Autodesk Fusion 360 part; units mm, degrees
(part 7 of 7)
  spline S38 degree 5 poles (-2.0348, 11.0912) (-2.0357, 11.0961) (-2.0377, 11.106) (-2.041, 11.1207) (-2.046, 11.1401) (-2.0533, 11.1642) (-2.0612, 11.1881) (-2.0696, 11.2119) (-2.0783, 11.2357) (-2.0871, 11.2594) (-2.096, 11.2831) (-2.1052, 11.3068) (-2.1147, 11.3304) (-2.1244, 11.3539) (-2.1346, 11.3774) (-2.145, 11.4007) (-2.1557, 11.424) (-2.1666, 11.4472) (-2.1777, 11.4704) (-2.189, 11.4935) (-2.2005, 11.5166) (-2.2122, 11.5397) (-2.2241, 11.5626) (-2.2361, 11.5855) (-2.2484, 11.6084) (-2.2609, 11.6312) (-2.2736, 11.654) (-2.2864, 11.6767) (-2.2995, 11.6993) (-2.3126, 11.7219) (-2.326, 11.7444) (-2.3395, 11.7669) (-2.3532, 11.7894) (-2.3671, 11.8118) (-2.3811, 11.8341) (-2.3953, 11.8564) (-2.4096, 11.8786) (-2.4241, 11.9008) (-2.4387, 11.9229) (-2.4535, 11.945) (-2.4685, 11.967) (-2.4836, 11.989) (-2.4988, 12.011) (-2.5142, 12.0328) (-2.5297, 12.0547) (-2.5454, 12.0764) (-2.5612, 12.0982) (-2.5771, 12.1198) (-2.5932, 12.1415) (-2.6094, 12.163) (-2.6258, 12.1846) (-2.6423, 12.206) (-2.6589, 12.2274) (-2.6756, 12.2488) (-2.6925, 12.2701) (-2.7095, 12.2914) (-2.7267, 12.3126) (-2.744, 12.3338) (-2.7614, 12.3549) (-2.7789, 12.3759) (-2.7965, 12.3969) (-2.8143, 12.4179) (-2.8322, 12.4388) (-2.8502, 12.4596) (-2.8684, 12.4804) (-2.8866, 12.5012) (-2.905, 12.5219) (-2.9235, 12.5425) (-2.9421, 12.5631) (-2.9609, 12.5836) (-2.9797, 12.6041) (-2.9949, 12.6204) (-3.0064, 12.6327) (-3.014, 12.6408) (-3.0178, 12.6449) knots 0 0 0 0 0 0 0.01428571 0.02857143 0.04285714 0.05714286 0.07142857 0.08571429 0.1 0.11428571 0.12857143 0.14285714 0.15714286 0.17142857 0.18571429 0.2 0.21428571 0.22857143 0.24285714 0.25714286 0.27142857 0.28571429 0.3 0.31428571 0.32857143 0.34285714 0.35714286 0.37142857 0.38571429 0.4 0.41428571 0.42857143 0.44285714 0.45714286 0.47142857 0.48571429 0.5 0.51428571 0.52857143 0.54285714 0.55714286 0.57142857 0.58571429 0.6 0.61428571 0.62857143 0.64285714 0.65714286 0.67142857 0.68571429 0.7 0.71428571 0.72857143 0.74285714 0.75714286 0.77142857 0.78571429 0.8 0.81428571 0.82857143 0.84285714 0.85714286 0.87142857 0.88571429 0.9 0.91428571 0.92857143 0.94285714 0.95714286 0.97142857 0.98571429 1 1 1 1 1 1
  arc A39 (-3.0178, 12.6449) -> (-3.7089, 12.4597) centre (0, 0) ccw
  spline S39 degree 5 poles (-3.7089, 12.4597) (-3.7102, 12.4543) (-3.7127, 12.4434) (-3.7165, 12.4271) (-3.7215, 12.4053) (-3.7276, 12.3782) (-3.7336, 12.351) (-3.7394, 12.3239) (-3.7451, 12.2968) (-3.7507, 12.2696) (-3.7561, 12.2426) (-3.7614, 12.2155) (-3.7666, 12.1884) (-3.7717, 12.1614) (-3.7766, 12.1343) (-3.7814, 12.1073) (-3.786, 12.0803) (-3.7905, 12.0533) (-3.7949, 12.0264) (-3.7992, 11.9994) (-3.8033, 11.9725) (-3.8072, 11.9456) (-3.8111, 11.9187) (-3.8147, 11.8919) (-3.8183, 11.865) (-3.8217, 11.8382) (-3.825, 11.8114) (-3.8281, 11.7846) (-3.831, 11.7579) (-3.8339, 11.7312) (-3.8365, 11.7045) (-3.8391, 11.6778) (-3.8415, 11.6512) (-3.8437, 11.6246) (-3.8458, 11.598) (-3.8477, 11.5714) (-3.8495, 11.5449) (-3.8511, 11.5184) (-3.8525, 11.492) (-3.8538, 11.4656) (-3.855, 11.4392) (-3.8559, 11.4128) (-3.8567, 11.3865) (-3.8574, 11.3602) (-3.8578, 11.334) (-3.8581, 11.3078) (-3.8583, 11.2816) (-3.8582, 11.2555) (-3.858, 11.2294) (-3.8576, 11.2034) (-3.857, 11.1774) (-3.8562, 11.1514) (-3.8552, 11.1256) (-3.854, 11.0997) (-3.8526, 11.0739) (-3.851, 11.0482) (-3.8492, 11.0225) (-3.8473, 10.9969) (-3.8451, 10.9713) (-3.8427, 10.9458) (-3.8401, 10.9204) (-3.8371, 10.895) (-3.8339, 10.8698) (-3.8302, 10.8446) (-3.8264, 10.8195) (-3.8223, 10.7945) (-3.818, 10.7695) (-3.8136, 10.7446) (-3.809, 10.7198) (-3.8039, 10.6951) (-3.7981, 10.6706) (-3.7928, 10.6513) (-3.7883, 10.6369) (-3.7851, 10.6274) (-3.7834, 10.6227) knots -1 -1 -1 -1 -1 -1 -0.98571429 -0.97142857 -0.95714286 -0.94285714 -0.92857143 -0.91428571 -0.9 -0.88571429 -0.87142857 -0.85714286 -0.84285714 -0.82857143 -0.81428571 -0.8 -0.78571429 -0.77142857 -0.75714286 -0.74285714 -0.72857143 -0.71428571 -0.7 -0.68571429 -0.67142857 -0.65714286 -0.64285714 -0.62857143 -0.61428571 -0.6 -0.58571429 -0.57142857 -0.55714286 -0.54285714 -0.52857143 -0.51428571 -0.5 -0.48571429 -0.47142857 -0.45714286 -0.44285714 -0.42857143 -0.41428571 -0.4 -0.38571429 -0.37142857 -0.35714286 -0.34285714 -0.32857143 -0.31428571 -0.3 -0.28571429 -0.27142857 -0.25714286 -0.24285714 -0.22857143 -0.21428571 -0.2 -0.18571429 -0.17142857 -0.15714286 -0.14285714 -0.12857143 -0.11428571 -0.1 -0.08571429 -0.07142857 -0.05714286 -0.04285714 -0.02857143 -0.01428571 0 0 0 0 0 0
  line L43 (-3.7834, 10.6227) -> (-3.6073, 10.1259)
  arc A40 (-3.6073, 10.1259) -> (-4.6093, 9.7108) centre (0, 0) ccw
  line L44 (-4.6093, 9.7108) -> (-4.8361, 10.1866)
  spline S40 degree 5 poles (-4.8361, 10.1866) (-4.8383, 10.1912) (-4.8427, 10.2002) (-4.8497, 10.2135) (-4.8596, 10.231) (-4.8728, 10.2523) (-4.8867, 10.2734) (-4.901, 10.2942) (-4.9155, 10.315) (-4.9301, 10.3356) (-4.9449, 10.3562) (-4.9599, 10.3767) (-4.9751, 10.397) (-4.9907, 10.4172) (-5.0065, 10.4372) (-5.0226, 10.4571) (-5.039, 10.4768) (-5.0555, 10.4964) (-5.0723, 10.5159) (-5.0892, 10.5353) (-5.1063, 10.5547) (-5.1235, 10.5739) (-5.1409, 10.593) (-5.1585, 10.612) (-5.1763, 10.6309) (-5.1942, 10.6497) (-5.2124, 10.6684) (-5.2307, 10.687) (-5.2491, 10.7055) (-5.2677, 10.7239) (-5.2864, 10.7422) (-5.3053, 10.7605) (-5.3243, 10.7786) (-5.3435, 10.7966) (-5.3628, 10.8146) (-5.3823, 10.8324) (-5.4019, 10.8502) (-5.4216, 10.8679) (-5.4415, 10.8855) (-5.4615, 10.903) (-5.4817, 10.9204) (-5.5019, 10.9377) (-5.5223, 10.955) (-5.5428, 10.9721) (-5.5635, 10.9892) (-5.5842, 11.0062) (-5.6051, 11.023) (-5.6261, 11.0399) (-5.6473, 11.0566) (-5.6685, 11.0732) (-5.6899, 11.0898) (-5.7114, 11.1062) (-5.733, 11.1226) (-5.7547, 11.1389) (-5.7765, 11.1552) (-5.7985, 11.1713) (-5.8205, 11.1873) (-5.8427, 11.2033) (-5.8649, 11.2192) (-5.8873, 11.235) (-5.9098, 11.2507) (-5.9324, 11.2664) (-5.9551, 11.2819) (-5.9779, 11.2974) (-6.0008, 11.3128) (-6.0238, 11.3281) (-6.0469, 11.3433) (-6.0701, 11.3585) (-6.0935, 11.3735) (-6.1169, 11.3885) (-6.1404, 11.4034) (-6.1593, 11.4153) (-6.1735, 11.4241) (-6.183, 11.43) (-6.1877, 11.4329) knots 0 0 0 0 0 0 0.01428571 0.02857143 0.04285714 0.05714286 0.07142857 0.08571429 0.1 0.11428571 0.12857143 0.14285714 0.15714286 0.17142857 0.18571429 0.2 0.21428571 0.22857143 0.24285714 0.25714286 0.27142857 0.28571429 0.3 0.31428571 0.32857143 0.34285714 0.35714286 0.37142857 0.38571429 0.4 0.41428571 0.42857143 0.44285714 0.45714286 0.47142857 0.48571429 0.5 0.51428571 0.52857143 0.54285714 0.55714286 0.57142857 0.58571429 0.6 0.61428571 0.62857143 0.64285714 0.65714286 0.67142857 0.68571429 0.7 0.71428571 0.72857143 0.74285714 0.75714286 0.77142857 0.78571429 0.8 0.81428571 0.82857143 0.84285714 0.85714286 0.87142857 0.88571429 0.9 0.91428571 0.92857143 0.94285714 0.95714286 0.97142857 0.98571429 1 1 1 1 1 1
  arc A41 (-6.1877, 11.4329) -> (-6.8073, 11.0752) centre (0, 0) ccw
  spline S41 degree 5 poles (-6.8073, 11.0752) (-6.8072, 11.0696) (-6.8068, 11.0585) (-6.8063, 11.0417) (-6.8054, 11.0194) (-6.8043, 10.9916) (-6.803, 10.9638) (-6.8016, 10.9361) (-6.8001, 10.9085) (-6.7985, 10.8808) (-6.7967, 10.8532) (-6.7949, 10.8257) (-6.7929, 10.7982) (-6.7908, 10.7708) (-6.7885, 10.7434) (-6.7861, 10.7161) (-6.7836, 10.6888) (-6.781, 10.6616) (-6.7783, 10.6344) (-6.7754, 10.6073) (-6.7724, 10.5802) (-6.7693, 10.5532) (-6.766, 10.5262) (-6.7626, 10.4993) (-6.7591, 10.4725) (-6.7554, 10.4457) (-6.7516, 10.419) (-6.7477, 10.3923) (-6.7437, 10.3657) (-6.7395, 10.3392) (-6.7352, 10.3127) (-6.7307, 10.2863) (-6.7261, 10.2599) (-6.7214, 10.2337) (-6.7165, 10.2074) (-6.7115, 10.1813) (-6.7063, 10.1552) (-6.701, 10.1292) (-6.6956, 10.1033) (-6.69, 10.0774) (-6.6843, 10.0516) (-6.6784, 10.0259) (-6.6724, 10.0003) (-6.6662, 9.9748) (-6.6598, 9.9493) (-6.6533, 9.9239) (-6.6467, 9.8986) (-6.6399, 9.8734) (-6.6329, 9.8483) (-6.6258, 9.8232) (-6.6185, 9.7983) (-6.611, 9.7734) (-6.6034, 9.7487) (-6.5955, 9.724) (-6.5875, 9.6995) (-6.5793, 9.675) (-6.5709, 9.6507) (-6.5624, 9.6264) (-6.5537, 9.6023) (-6.5448, 9.5783) (-6.5356, 9.5544) (-6.5262, 9.5307) (-6.5165, 9.5071) (-6.5065, 9.4837) (-6.4963, 9.4605) (-6.4859, 9.4374) (-6.4753, 9.4144) (-6.4646, 9.3915) (-6.4537, 9.3687) (-6.4424, 9.3462) (-6.4305, 9.324) (-6.4203, 9.3067) (-6.4123, 9.294) (-6.4067, 9.2856) (-6.4038, 9.2815) knots -1 -1 -1 -1 -1 -1 -0.98571429 -0.97142857 -0.95714286 -0.94285714 -0.92857143 -0.91428571 -0.9 -0.88571429 -0.87142857 -0.85714286 -0.84285714 -0.82857143 -0.81428571 -0.8 -0.78571429 -0.77142857 -0.75714286 -0.74285714 -0.72857143 -0.71428571 -0.7 -0.68571429 -0.67142857 -0.65714286 -0.64285714 -0.62857143 -0.61428571 -0.6 -0.58571429 -0.57142857 -0.55714286 -0.54285714 -0.52857143 -0.51428571 -0.5 -0.48571429 -0.47142857 -0.45714286 -0.44285714 -0.42857143 -0.41428571 -0.4 -0.38571429 -0.37142857 -0.35714286 -0.34285714 -0.32857143 -0.31428571 -0.3 -0.28571429 -0.27142857 -0.25714286 -0.24285714 -0.22857143 -0.21428571 -0.2 -0.18571429 -0.17142857 -0.15714286 -0.14285714 -0.12857143 -0.11428571 -0.1 -0.08571429 -0.07142857 -0.05714286 -0.04285714 -0.02857143 -0.01428571 0 0 0 0 0 0
  line L45 (-6.4038, 9.2815) -> (-6.1051, 8.8472)
  arc A42 (-6.1051, 8.8472) -> (-6.9656, 8.1869) centre (0, 0) ccw
  line L46 (-6.9656, 8.1869) -> (-7.3078, 8.5878)
  spline S42 degree 5 poles (-7.3078, 8.5878) (-7.3111, 8.5917) (-7.3177, 8.5992) (-7.3279, 8.6103) (-7.342, 8.6246) (-7.3603, 8.6418) (-7.3791, 8.6586) (-7.3983, 8.675) (-7.4177, 8.6913) (-7.4372, 8.7074) (-7.4568, 8.7235) (-7.4766, 8.7394) (-7.4966, 8.7551) (-7.5168, 8.7706) (-7.5373, 8.7858) (-7.558, 8.8008) (-7.5789, 8.8156) (-7.6, 8.8303) (-7.6212, 8.8448) (-7.6425, 8.8592) (-7.664, 8.8734) (-7.6856, 8.8875) (-7.7074, 8.9015) (-7.7293, 8.9153) (-7.7514, 8.929) (-7.7736, 8.9425) (-7.796, 8.9558) (-7.8184, 8.9691) (-7.841, 8.9822) (-7.8638, 8.9951) (-7.8866, 9.008) (-7.9096, 9.0207) (-7.9326, 9.0333) (-7.9558, 9.0457) (-7.9791, 9.0581) (-8.0025, 9.0703) (-8.0261, 9.0824) (-8.0497, 9.0943) (-8.0735, 9.1062) (-8.0973, 9.1179) (-8.1213, 9.1295) (-8.1453, 9.141) (-8.1695, 9.1524) (-8.1938, 9.1637) (-8.2181, 9.1748) (-8.2426, 9.1858) (-8.2671, 9.1967) (-8.2918, 9.2075) (-8.3165, 9.2182) (-8.3413, 9.2288) (-8.3663, 9.2392) (-8.3913, 9.2496) (-8.4164, 9.2598) (-8.4416, 9.27) (-8.4669, 9.28) (-8.4922, 9.2899) (-8.5177, 9.2997) (-8.5432, 9.3094) (-8.5688, 9.319) (-8.5945, 9.3284) (-8.6203, 9.3378) (-8.6462, 9.347) (-8.6722, 9.3562) (-8.6982, 9.3652) (-8.7243, 9.3742) (-8.7505, 9.383) (-8.7768, 9.3917) (-8.8031, 9.4004) (-8.8295, 9.4089) (-8.856, 9.4173) (-8.8826, 9.4256) (-8.9039, 9.4321) (-8.9199, 9.437) (-8.9306, 9.4403) (-8.936, 9.4419) knots 0 0 0 0 0 0 0.01428571 0.02857143 0.04285714 0.05714286 0.07142857 0.08571429 0.1 0.11428571 0.12857143 0.14285714 0.15714286 0.17142857 0.18571429 0.2 0.21428571 0.22857143 0.24285714 0.25714286 0.27142857 0.28571429 0.3 0.31428571 0.32857143 0.34285714 0.35714286 0.37142857 0.38571429 0.4 0.41428571 0.42857143 0.44285714 0.45714286 0.47142857 0.48571429 0.5 0.51428571 0.52857143 0.54285714 0.55714286 0.57142857 0.58571429 0.6 0.61428571 0.62857143 0.64285714 0.65714286 0.67142857 0.68571429 0.7 0.71428571 0.72857143 0.74285714 0.75714286 0.77142857 0.78571429 0.8 0.81428571 0.82857143 0.84285714 0.85714286 0.87142857 0.88571429 0.9 0.91428571 0.92857143 0.94285714 0.95714286 0.97142857 0.98571429 1 1 1 1 1 1
  arc A43 (-8.936, 9.4419) -> (-9.4419, 8.936) centre (0, 0) ccw
  spline S43 degree 5 poles (-9.4419, 8.936) (-9.4403, 8.9306) (-9.437, 8.9199) (-9.4321, 8.9039) (-9.4256, 8.8826) (-9.4173, 8.856) (-9.4089, 8.8295) (-9.4004, 8.8031) (-9.3917, 8.7768) (-9.383, 8.7505) (-9.3742, 8.7243) (-9.3652, 8.6982) (-9.3562, 8.6722) (-9.347, 8.6462) (-9.3378, 8.6203) (-9.3284, 8.5945) (-9.319, 8.5688) (-9.3094, 8.5432) (-9.2997, 8.5177) (-9.2899, 8.4922) (-9.28, 8.4669) (-9.27, 8.4416) (-9.2598, 8.4164) (-9.2496, 8.3913) (-9.2392, 8.3663) (-9.2288, 8.3413) (-9.2182, 8.3165) (-9.2075, 8.2918) (-9.1967, 8.2671) (-9.1858, 8.2426) (-9.1748, 8.2181) (-9.1637, 8.1938) (-9.1524, 8.1695) (-9.141, 8.1453) (-9.1295, 8.1213) (-9.1179, 8.0973) (-9.1062, 8.0735) (-9.0943, 8.0497) (-9.0824, 8.0261) (-9.0703, 8.0025) (-9.0581, 7.9791) (-9.0457, 7.9558) (-9.0333, 7.9326) (-9.0207, 7.9096) (-9.008, 7.8866) (-8.9951, 7.8638) (-8.9822, 7.841) (-8.9691, 7.8184) (-8.9558, 7.796) (-8.9425, 7.7736) (-8.929, 7.7514) (-8.9153, 7.7293) (-8.9015, 7.7074) (-8.8875, 7.6856) (-8.8734, 7.664) (-8.8592, 7.6425) (-8.8448, 7.6212) (-8.8303, 7.6) (-8.8156, 7.5789) (-8.8008, 7.558) (-8.7858, 7.5373) (-8.7706, 7.5168) (-8.7551, 7.4966) (-8.7394, 7.4766) (-8.7235, 7.4568) (-8.7074, 7.4372) (-8.6913, 7.4177) (-8.675, 7.3983) (-8.6586, 7.3791) (-8.6418, 7.3603) (-8.6246, 7.342) (-8.6103, 7.3279) (-8.5992, 7.3177) (-8.5917, 7.3111) (-8.5878, 7.3078) knots -1 -1 -1 -1 -1 -1 -0.98571429 -0.97142857 -0.95714286 -0.94285714 -0.92857143 -0.91428571 -0.9 -0.88571429 -0.87142857 -0.85714286 -0.84285714 -0.82857143 -0.81428571 -0.8 -0.78571429 -0.77142857 -0.75714286 -0.74285714 -0.72857143 -0.71428571 -0.7 -0.68571429 -0.67142857 -0.65714286 -0.64285714 -0.62857143 -0.61428571 -0.6 -0.58571429 -0.57142857 -0.55714286 -0.54285714 -0.52857143 -0.51428571 -0.5 -0.48571429 -0.47142857 -0.45714286 -0.44285714 -0.42857143 -0.41428571 -0.4 -0.38571429 -0.37142857 -0.35714286 -0.34285714 -0.32857143 -0.31428571 -0.3 -0.28571429 -0.27142857 -0.25714286 -0.24285714 -0.22857143 -0.21428571 -0.2 -0.18571429 -0.17142857 -0.15714286 -0.14285714 -0.12857143 -0.11428571 -0.1 -0.08571429 -0.07142857 -0.05714286 -0.04285714 -0.02857143 -0.01428571 0 0 0 0 0 0
  line L47 (-8.5878, 7.3078) -> (-8.1869, 6.9656)
  arc A44 (-8.1869, 6.9656) -> (-8.8472, 6.1051) centre (0, 0) ccw
  line L48 (-8.8472, 6.1051) -> (-9.2815, 6.4038)
  spline S44 degree 5 poles (-9.2815, 6.4038) (-9.2856, 6.4067) (-9.294, 6.4123) (-9.3067, 6.4203) (-9.324, 6.4305) (-9.3462, 6.4424) (-9.3687, 6.4537) (-9.3915, 6.4646) (-9.4144, 6.4753) (-9.4374, 6.4859) (-9.4605, 6.4963) (-9.4837, 6.5065) (-9.5071, 6.5165) (-9.5307, 6.5262) (-9.5544, 6.5356) (-9.5783, 6.5448) (-9.6023, 6.5537) (-9.6264, 6.5624) (-9.6507, 6.5709) (-9.675, 6.5793) (-9.6995, 6.5875) (-9.724, 6.5955) (-9.7487, 6.6034) (-9.7734, 6.611) (-9.7983, 6.6185) (-9.8232, 6.6258) (-9.8483, 6.6329) (-9.8734, 6.6399) (-9.8986, 6.6467) (-9.9239, 6.6533) (-9.9493, 6.6598) (-9.9748, 6.6662) (-10.0003, 6.6724) (-10.0259, 6.6784) (-10.0516, 6.6843) (-10.0774, 6.69) (-10.1033, 6.6956) (-10.1292, 6.701) (-10.1552, 6.7063) (-10.1813, 6.7115) (-10.2074, 6.7165) (-10.2337, 6.7214) (-10.2599, 6.7261) (-10.2863, 6.7307) (-10.3127, 6.7352) (-10.3392, 6.7395) (-10.3657, 6.7437) (-10.3923, 6.7477) (-10.419, 6.7516) (-10.4457, 6.7554) (-10.4725, 6.7591) (-10.4993, 6.7626) (-10.5262, 6.766) (-10.5532, 6.7693) (-10.5802, 6.7724) (-10.6073, 6.7754) (-10.6344, 6.7783) (-10.6616, 6.781) (-10.6888, 6.7836) (-10.7161, 6.7861) (-10.7434, 6.7885) (-10.7708, 6.7908) (-10.7982, 6.7929) (-10.8257, 6.7949) (-10.8532, 6.7967) (-10.8808, 6.7985) (-10.9085, 6.8001) (-10.9361, 6.8016) (-10.9638, 6.803) (-10.9916, 6.8043) (-11.0194, 6.8054) (-11.0417, 6.8063) (-11.0585, 6.8068) (-11.0696, 6.8072) (-11.0752, 6.8073) knots 0 0 0 0 0 0 0.01428571 0.02857143 0.04285714 0.05714286 0.07142857 0.08571429 0.1 0.11428571 0.12857143 0.14285714 0.15714286 0.17142857 0.18571429 0.2 0.21428571 0.22857143 0.24285714 0.25714286 0.27142857 0.28571429 0.3 0.31428571 0.32857143 0.34285714 0.35714286 0.37142857 0.38571429 0.4 0.41428571 0.42857143 0.44285714 0.45714286 0.47142857 0.48571429 0.5 0.51428571 0.52857143 0.54285714 0.55714286 0.57142857 0.58571429 0.6 0.61428571 0.62857143 0.64285714 0.65714286 0.67142857 0.68571429 0.7 0.71428571 0.72857143 0.74285714 0.75714286 0.77142857 0.78571429 0.8 0.81428571 0.82857143 0.84285714 0.85714286 0.87142857 0.88571429 0.9 0.91428571 0.92857143 0.94285714 0.95714286 0.97142857 0.98571429 1 1 1 1 1 1
  arc A45 (-11.0752, 6.8073) -> (-11.4329, 6.1877) centre (0, 0) ccw
  spline S45 degree 5 poles (-11.4329, 6.1877) (-11.43, 6.183) (-11.4241, 6.1735) (-11.4153, 6.1593) (-11.4034, 6.1404) (-11.3885, 6.1169) (-11.3735, 6.0935) (-11.3585, 6.0701) (-11.3433, 6.0469) (-11.3281, 6.0238) (-11.3128, 6.0008) (-11.2974, 5.9779) (-11.2819, 5.9551) (-11.2664, 5.9324) (-11.2507, 5.9098) (-11.235, 5.8873) (-11.2192, 5.8649) (-11.2033, 5.8427) (-11.1873, 5.8205) (-11.1713, 5.7985) (-11.1552, 5.7765) (-11.1389, 5.7547) (-11.1226, 5.733) (-11.1062, 5.7114) (-11.0898, 5.6899) (-11.0732, 5.6685) (-11.0566, 5.6473) (-11.0399, 5.6261) (-11.023, 5.6051) (-11.0062, 5.5842) (-10.9892, 5.5635) (-10.9721, 5.5428) (-10.955, 5.5223) (-10.9377, 5.5019) (-10.9204, 5.4817) (-10.903, 5.4615) (-10.8855, 5.4415) (-10.8679, 5.4216) (-10.8502, 5.4019) (-10.8324, 5.3823) (-10.8146, 5.3628) (-10.7966, 5.3435) (-10.7786, 5.3243) (-10.7605, 5.3053) (-10.7422, 5.2864) (-10.7239, 5.2677) (-10.7055, 5.2491) (-10.687, 5.2307) (-10.6684, 5.2124) (-10.6497, 5.1942) (-10.6309, 5.1763) (-10.612, 5.1585) (-10.593, 5.1409) (-10.5739, 5.1235) (-10.5547, 5.1063) (-10.5353, 5.0892) (-10.5159, 5.0723) (-10.4964, 5.0555) (-10.4768, 5.039) (-10.4571, 5.0226) (-10.4372, 5.0065) (-10.4172, 4.9907) (-10.397, 4.9751) (-10.3767, 4.9599) (-10.3562, 4.9449) (-10.3356, 4.9301) (-10.315, 4.9155) (-10.2942, 4.901) (-10.2734, 4.8867) (-10.2523, 4.8728) (-10.231, 4.8596) (-10.2135, 4.8497) (-10.2002, 4.8427) (-10.1912, 4.8383) (-10.1866, 4.8361) knots -1 -1 -1 -1 -1 -1 -0.98571429 -0.97142857 -0.95714286 -0.94285714 -0.92857143 -0.91428571 -0.9 -0.88571429 -0.87142857 -0.85714286 -0.84285714 -0.82857143 -0.81428571 -0.8 -0.78571429 -0.77142857 -0.75714286 -0.74285714 -0.72857143 -0.71428571 -0.7 -0.68571429 -0.67142857 -0.65714286 -0.64285714 -0.62857143 -0.61428571 -0.6 -0.58571429 -0.57142857 -0.55714286 -0.54285714 -0.52857143 -0.51428571 -0.5 -0.48571429 -0.47142857 -0.45714286 -0.44285714 -0.42857143 -0.41428571 -0.4 -0.38571429 -0.37142857 -0.35714286 -0.34285714 -0.32857143 -0.31428571 -0.3 -0.28571429 -0.27142857 -0.25714286 -0.24285714 -0.22857143 -0.21428571 -0.2 -0.18571429 -0.17142857 -0.15714286 -0.14285714 -0.12857143 -0.11428571 -0.1 -0.08571429 -0.07142857 -0.05714286 -0.04285714 -0.02857143 -0.01428571 0 0 0 0 0 0
  line L49 (-10.1866, 4.8361) -> (-9.7108, 4.6093)
  arc A46 (-9.7108, 4.6093) -> (-10.1259, 3.6073) centre (0, 0) ccw
  line L50 (-10.1259, 3.6073) -> (-10.6227, 3.7834)
  spline S46 degree 5 poles (-10.6227, 3.7834) (-10.6274, 3.7851) (-10.6369, 3.7883) (-10.6513, 3.7928) (-10.6706, 3.7981) (-10.6951, 3.8039) (-10.7198, 3.809) (-10.7446, 3.8136) (-10.7695, 3.818) (-10.7945, 3.8223) (-10.8195, 3.8264) (-10.8446, 3.8302) (-10.8698, 3.8339) (-10.895, 3.8371) (-10.9204, 3.8401) (-10.9458, 3.8427) (-10.9713, 3.8451) (-10.9969, 3.8473) (-11.0225, 3.8492) (-11.0482, 3.851) (-11.0739, 3.8526) (-11.0997, 3.854) (-11.1256, 3.8552) (-11.1514, 3.8562) (-11.1774, 3.857) (-11.2034, 3.8576) (-11.2294, 3.858) (-11.2555, 3.8582) (-11.2816, 3.8583) (-11.3078, 3.8581) (-11.334, 3.8578) (-11.3602, 3.8574) (-11.3865, 3.8567) (-11.4128, 3.8559) (-11.4392, 3.855) (-11.4656, 3.8538) (-11.492, 3.8525) (-11.5184, 3.8511) (-11.5449, 3.8495) (-11.5714, 3.8477) (-11.598, 3.8458) (-11.6246, 3.8437) (-11.6512, 3.8415) (-11.6778, 3.8391) (-11.7045, 3.8365) (-11.7312, 3.8339) (-11.7579, 3.831) (-11.7846, 3.8281) (-11.8114, 3.825) (-11.8382, 3.8217) (-11.865, 3.8183) (-11.8919, 3.8147) (-11.9187, 3.8111) (-11.9456, 3.8072) (-11.9725, 3.8033) (-11.9994, 3.7992) (-12.0264, 3.7949) (-12.0533, 3.7905) (-12.0803, 3.786) (-12.1073, 3.7814) (-12.1343, 3.7766) (-12.1614, 3.7717) (-12.1884, 3.7666) (-12.2155, 3.7614) (-12.2426, 3.7561) (-12.2696, 3.7507) (-12.2968, 3.7451) (-12.3239, 3.7394) (-12.351, 3.7336) (-12.3782, 3.7276) (-12.4053, 3.7215) (-12.4271, 3.7165) (-12.4434, 3.7127) (-12.4543, 3.7102) (-12.4597, 3.7089) knots 0 0 0 0 0 0 0.01428571 0.02857143 0.04285714 0.05714286 0.07142857 0.08571429 0.1 0.11428571 0.12857143 0.14285714 0.15714286 0.17142857 0.18571429 0.2 0.21428571 0.22857143 0.24285714 0.25714286 0.27142857 0.28571429 0.3 0.31428571 0.32857143 0.34285714 0.35714286 0.37142857 0.38571429 0.4 0.41428571 0.42857143 0.44285714 0.45714286 0.47142857 0.48571429 0.5 0.51428571 0.52857143 0.54285714 0.55714286 0.57142857 0.58571429 0.6 0.61428571 0.62857143 0.64285714 0.65714286 0.67142857 0.68571429 0.7 0.71428571 0.72857143 0.74285714 0.75714286 0.77142857 0.78571429 0.8 0.81428571 0.82857143 0.84285714 0.85714286 0.87142857 0.88571429 0.9 0.91428571 0.92857143 0.94285714 0.95714286 0.97142857 0.98571429 1 1 1 1 1 1
  arc A47 (-12.4597, 3.7089) -> (-12.6449, 3.0178) centre (0, 0) ccw
  spline S47 degree 5 poles (-12.6449, 3.0178) (-12.6408, 3.014) (-12.6327, 3.0064) (-12.6204, 2.9949) (-12.6041, 2.9797) (-12.5836, 2.9609) (-12.5631, 2.9421) (-12.5425, 2.9235) (-12.5219, 2.905) (-12.5012, 2.8866) (-12.4804, 2.8684) (-12.4596, 2.8502) (-12.4388, 2.8322) (-12.4179, 2.8143) (-12.3969, 2.7965) (-12.3759, 2.7789) (-12.3549, 2.7614) (-12.3338, 2.744) (-12.3126, 2.7267) (-12.2914, 2.7095) (-12.2701, 2.6925) (-12.2488, 2.6756) (-12.2274, 2.6589) (-12.206, 2.6423) (-12.1846, 2.6258) (-12.163, 2.6094) (-12.1415, 2.5932) (-12.1198, 2.5771) (-12.0982, 2.5612) (-12.0764, 2.5454) (-12.0547, 2.5297) (-12.0328, 2.5142) (-12.011, 2.4988) (-11.989, 2.4836) (-11.967, 2.4685) (-11.945, 2.4535) (-11.9229, 2.4387) (-11.9008, 2.4241) (-11.8786, 2.4096) (-11.8564, 2.3953) (-11.8341, 2.3811) (-11.8118, 2.3671) (-11.7894, 2.3532) (-11.7669, 2.3395) (-11.7444, 2.326) (-11.7219, 2.3126) (-11.6993, 2.2995) (-11.6767, 2.2864) (-11.654, 2.2736) (-11.6312, 2.2609) (-11.6084, 2.2484) (-11.5855, 2.2361) (-11.5626, 2.2241) (-11.5397, 2.2122) (-11.5166, 2.2005) (-11.4935, 2.189) (-11.4704, 2.1777) (-11.4472, 2.1666) (-11.424, 2.1557) (-11.4007, 2.145) (-11.3774, 2.1346) (-11.3539, 2.1244) (-11.3304, 2.1147) (-11.3068, 2.1052) (-11.2831, 2.096) (-11.2594, 2.0871) (-11.2357, 2.0783) (-11.2119, 2.0696) (-11.1881, 2.0612) (-11.1642, 2.0533) (-11.1401, 2.046) (-11.1207, 2.041) (-11.106, 2.0377) (-11.0961, 2.0357) (-11.0912, 2.0348) knots -1 -1 -1 -1 -1 -1 -0.98571429 -0.97142857 -0.95714286 -0.94285714 -0.92857143 -0.91428571 -0.9 -0.88571429 -0.87142857 -0.85714286 -0.84285714 -0.82857143 -0.81428571 -0.8 -0.78571429 -0.77142857 -0.75714286 -0.74285714 -0.72857143 -0.71428571 -0.7 -0.68571429 -0.67142857 -0.65714286 -0.64285714 -0.62857143 -0.61428571 -0.6 -0.58571429 -0.57142857 -0.55714286 -0.54285714 -0.52857143 -0.51428571 -0.5 -0.48571429 -0.47142857 -0.45714286 -0.44285714 -0.42857143 -0.41428571 -0.4 -0.38571429 -0.37142857 -0.35714286 -0.34285714 -0.32857143 -0.31428571 -0.3 -0.28571429 -0.27142857 -0.25714286 -0.24285714 -0.22857143 -0.21428571 -0.2 -0.18571429 -0.17142857 -0.15714286 -0.14285714 -0.12857143 -0.11428571 -0.1 -0.08571429 -0.07142857 -0.05714286 -0.04285714 -0.02857143 -0.01428571 0 0 0 0 0 0
  line L51 (-11.0912, 2.0348) -> (-10.5729, 1.9389)
  circle A48 centre (0, 0) radius 4
  dimension "d40" = 8
  constraint coincident A0.centre A1.centre
  measures "d40" diameter of A48
extrude "Extrude4" add sketch "Sketch4" along normal blind 70 contours L0 L1 L2 L3 | A48 bodies 1 in component "Spur Gear (24 teeth) (1)"
sketch "Sketch5" plane through (0, 0, 0) normal (0, 0, 1) x (1, 0, 0)
  circle A0 centre (31.4681, -0.0658) radius 2.5
  circle A1 centre (31.4681, -0.0658) radius 7.5
  dimension "d43" = 5
  dimension "d44" = 15
  constraint concentric A0 A1
  measures "d43" diameter of A0
  measures "d44" diameter of A1
extrude "Extrude1'''" add sketch "Sketch5" along normal blind 40 separate body makes body 3
copy_body "CopyPasteBodies1" bodies 3 makes body 4
move_body "Move1" bodies 4 to x (1, 0, 0) y (0, 1, 0) z (0, 0, 1) at (20, 0, 0)
sketch "Sketch6" plane through (0, 0, 0) normal (0, 0, 1) x (1, 0, 0)
  circle A0 centre (-0.3347, 41.8436) radius 4
  circle A1 centre (-0.3347, 41.8436) radius 7.5
  dimension "d47" = 8
  dimension "d48" = 15
  constraint concentric A0 A1
  measures "d47" diameter of A0
  measures "d48" diameter of A1
extrude "Extrude2'''" add sketch "Sketch6" along normal blind 30 separate body makes body 5
component "Spur Gear (24 teeth) (1)" placed x (1, 0, 0) y (0, 1, 0) z (0, 0, 1) at (0, 0, 0)
component "Spur Gear (12 teeth)" placed x (1, 0, 0) y (0, 1, 0) z (0, 0, 1) at (0, 0, 0)
component "Spur Gear (12 teeth) (1)" placed x (1, 0, 0) y (0, 1, 0) z (0, 0, 1) at (-8.2967, -24.6131, -3.0566)
component "Spur Gear (12 teeth) (1)" placed x (1, 0, 0) y (0, 1, 0) z (0, 0, 1) at (11.1532, -22.9, -3.8414)
hidden bodies 3 4 5
